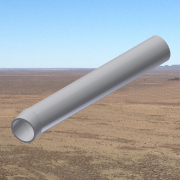
# Autodesk Inventor part: 2r2scs
Saved by Autodesk Inventor 2014 SP1 (Build 180222100, 222)
## iProperties
Company: HERA Project
Created: 2013-06-11
Part Number: 2r2scs
Material: PVC-Piping
Document SubType Name: Modeling
Designer: David DeBoer
Density: 1.4 g/cm^3
Description: spar cross support holder
Mass: 468.384 g
Surface Area: 1724.47 cm^2
Volume: 334.56 cm^3
Appearance: Smooth - White
Author: David DeBoer
Title: Hub-supporthold
Autodesk Inventor part; units mm, degrees
ref_plane "YZ Plane" through (0, 0, 0) normal (1, 0, 0) x (0, 1, 0)
ref_plane "XZ Plane" through (0, 0, 0) normal (0, 1, 0) x (-1, 0, 0)
sketch "Sketch1" plane through (0, 0, 0) normal (0, 0, 1) x (1, 0, 0)
  circle A0 centre (0, 0) radius 30.1625
  circle A1 centre (0, 0) radius 26.2509
  dimension "d0" = 60.325
  dimension "d2" = 3.9116
  constraints: 2 centre point, 1 coincident
  measures "d0" diameter of A0
  measures "d2" radial gap between concentric circles of A1 A0
extrude "Extrusion1" add sketch "Sketch1" along normal blind 381
sketch "Sketch16" plane through (0, 0, 381) normal (0, 0, 1) x (1, 0, 0)
  circle A0 centre (0, 0) radius 30.1625 projected
  line L0 (27.5395, -2.4255) -> (30.1625, -2.4255)
  line L1 (30.1625, -2.4255) -> (30.1625, 0)
  line L2 (30.1625, 0) -> (27.5395, 0)
  line L3 (27.5395, 0) -> (27.5395, -2.4255)
  constraints: 8 end point, 2 parallel, 1 horizontal, 1 horizontal alignment, 1 perpendicular, 1 other
extrude "Extrusion9" add sketch "Sketch16" along normal blind 0.254 contours L1 L0 A0 | A0 L0 L3 L2 picked at (28.3994, -1.3478)
ref_plane "Work Plane7" through (30.1625, -2.4255, 381.254) normal (0.258819, 0, 0.9659258) x (0, 1, 0)
sketch "Sketch17" plane through (30.1625, -2.4255, 381.254) normal (0.258819, 0, 0.9659258) x (0, 1, 0)
  circle A0 centre (2.4255, 29.9579) radius 30.1625
  circle A1 centre (2.4255, 29.9579) radius 26.2509
  point P0 (2.4255, -69.5411)
  dimension "d54" = 60.325
  dimension "d55" = 3.9116
  constraints: 2 centre point
  measures "d54" diameter of A0
  measures "d55" radial gap between concentric circles of A1 A0
extrude "Extrusion10" add sketch "Sketch17" along normal blind 25.4 draft 0.2 and the other way blind 15.24
body "Solid1"
